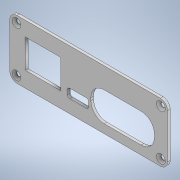
# Autodesk Inventor part: cover-slave
Saved by Autodesk Inventor 2021 (Build 250183000, 183)
## iProperties
Created: 2025-06-25
Part Number: cover-slave
Material: Generic
Document SubType Name: Modeling
Designer: Toby
Density: 1 g/cm^3
Appearance: Default
Author: Toby
Autodesk Inventor part; units mm, degrees
ref_plane "YZ Plane" through (0, 0, 0) normal (1, 0, 0) x (0, 1, 0)
ref_plane "XZ Plane" through (0, 0, 0) normal (0, 1, 0) x (-1, 0, 0)
ref_plane "XY Plane" through (0, 0, 0) normal (0, 0, 1) x (1, 0, 0)
sketch "Sketch1" plane through (0, 0, 0) normal (0, 0, 1) x (1, 0, 0)
  line L0 (-35.5, 13.25) -> (35.5, 13.25)
  line L1 (35.5, 13.25) -> (35.5, -13.25)
  line L2 (35.5, -13.25) -> (-35.5, -13.25)
  line L3 (-35.5, -13.25) -> (-35.5, 13.25)
  point P0 (0, 0)
  dimension "d0" = 26.5
  dimension "d1" = 71
  dimension "d2" = 35.5
  dimension "d3" = 13.25
  constraints: 8 end point, 2 parallel, 1 horizontal, 1 perpendicular
  measures "d0" distance of L2.end L0.start
  measures "d1" distance of L0.start L0.end
  measures "d2" distance from line of point (0, 0) L3
  measures "d3" distance from line of point (0, 0) L0
extrude "Extrusion1" add sketch "Sketch1" along normal blind 1.2
fillet "Fillet1" radius 3.25 4 edges at (-35.5, 13.25, 0.6) (-35.5, -13.25, 0.6) (35.5, -13.25, 0.6) (35.5, 13.25, 0.6)
sketch "Sketch2" plane through (0, 0, 1.2) normal (0, 0, 1) x (1, 0, 0)
  line L0 (32.25, 13.25) -> (-32.25, 13.25) projected
  line L1 (-35.5, 10) -> (-35.5, -10) projected
  line L2 (-32.25, -13.25) -> (32.25, -13.25) projected
  line L3 (35.5, -10) -> (35.5, 10) projected
  point P0 (0, 0)
  point P1 (-32.5, 10.25)
  point P2 (32.5, 10.25)
  point P3 (32.5, -10.25)
  point P4 (-32.5, -10.25)
  dimension "d7" = 3
  dimension "d8" = 3
  dimension "d9" = 3
  dimension "d10" = 3
  dimension "d11" = 3
  dimension "d12" = 3
  dimension "d13" = 3
  dimension "d14" = 3
  measures "d7" distance from line of L0 point (-32.5, 10.25)
  measures "d8" distance from line of L1 point (-32.5, 10.25)
  measures "d9" distance from line of L1 point (-32.5, -10.25)
  measures "d10" distance from line of L2 point (-32.5, -10.25)
  measures "d11" distance from line of L3 point (32.5, -10.25)
  measures "d12" distance from line of L2 point (32.5, -10.25)
  measures "d13" distance from line of L0 point (32.5, 10.25)
  measures "d14" distance from line of L3 point (32.5, 10.25)
hole "Hole1" at (-32.5, 10.25, 1.2) at (32.5, 10.25, 1.2) at (32.5, -10.25, 1.2) at (-32.5, -10.25, 1.2) direction (0, 0, -1) diameter 2 depth 4 tip angle 118 countersink diameter 4 countersink angle 90
sketch "Sketch3" plane through (0, 0, 1.2) normal (0, 0, 1) x (1, 0, 0)
  line L0 (-28.5, 6.75) -> (-12.5, 6.75)
  line L1 (-12.5, 6.75) -> (-12.5, -6.25)
  line L2 (-12.5, -6.25) -> (-28.5, -6.25)
  line L3 (-28.5, -6.25) -> (-28.5, 6.75)
  line L4 (-35.5, 10) -> (-35.5, -10) projected
  line L5 (-32.25, -13.25) -> (32.25, -13.25) projected
  point P0 (0, 0)
  dimension "d22" = 7
  dimension "d23" = 23
  dimension "d24" = 7
  dimension "d25" = 20
  constraints: 8 end point, 2 parallel, 1 horizontal, 1 perpendicular
  measures "d22" distance between parallel lines of L4 L3
  measures "d23" distance between parallel lines of L4 L1
  measures "d24" distance between parallel lines of L5 L2
  measures "d25" distance between parallel lines of L5 L0
extrude "Extrusion2" cut sketch "Sketch3" against normal blind 2
sketch "Sketch4" plane through (0, 0, 1.2) normal (0, 0, 1) x (1, 0, 0)
  line L0 (-9.5, -3.25) -> (0, -3.25)
  line L1 (0, -3.25) -> (0, -7.25)
  line L2 (0, -7.25) -> (-9.5, -7.25)
  line L3 (-9.5, -7.25) -> (-9.5, -3.25)
  line L4 (-35.5, 10) -> (-35.5, -10) projected
  line L5 (-32.25, -13.25) -> (32.25, -13.25) projected
  point P0 (0, 0)
  dimension "d28" = 26
  dimension "d29" = 35.5
  dimension "d30" = 6
  dimension "d31" = 10
  constraints: 8 end point, 2 parallel, 1 horizontal, 1 perpendicular
  measures "d28" distance between parallel lines of L4 L3
  measures "d29" distance between parallel lines of L4 L1
  measures "d30" distance between parallel lines of L5 L2
  measures "d31" distance between parallel lines of L5 L0
extrude "Extrusion3" cut sketch "Sketch4" against normal blind 2
sketch "Sketch5" plane through (0, 0, 1.2) normal (0, 0, 1) x (1, 0, 0)
  line L0 (6.5, 1.75) -> (24.5, 1.75)
  line L1 (24.5, 1.75) -> (24.5, -5.25)
  line L2 (24.5, -5.25) -> (6.5, -5.25)
  line L3 (6.5, -5.25) -> (6.5, 1.75)
  line L4 (35.5, -10) -> (35.5, 10) projected
  line L5 (-32.25, -13.25) -> (32.25, -13.25) projected
  point P0 (0, 0)
  dimension "d34" = 11
  dimension "d35" = 29
  dimension "d36" = 15
  dimension "d37" = 8
  constraints: 8 end point, 2 parallel, 1 horizontal, 1 perpendicular
  measures "d34" distance between parallel lines of L4 L1
  measures "d35" distance between parallel lines of L4 L3
  measures "d36" distance between parallel lines of L5 L0
  measures "d37" distance between parallel lines of L5 L2
extrude "Extrusion4" cut sketch "Sketch5" against normal blind 2
chamfer "Chamfer1" distance 2 angle 45 2 edges at (6.5, -5.25, 0.6) (24.5, -5.25, 0.6)
fillet "Fillet2" radius 1 4 edges at (-9.5, -3.25, 0.6) (-9.5, -7.25, 0.6) (0, -7.25, 0.6) (0, -3.25, 0.6)
sketch "Sketch7" plane through (0, 0, 1.2) normal (0, 0, 1) x (1, 0, 0)
  line L0 (1, 3.85) -> (29.6, 3.85)
  line L1 (29.6, 3.85) -> (29.6, -9.35)
  line L2 (29.6, -9.35) -> (1, -9.35)
  line L3 (1, -9.35) -> (1, 3.85)
  line L4 (-32.25, -13.25) -> (32.25, -13.25) projected
  line L5 (35.5, -10) -> (35.5, 10) projected
  point P0 (0, 0)
  dimension "d56" = 3.9
  dimension "d57" = 5.9
  dimension "d58" = 17.1
  dimension "d59" = 34.5
  constraints: 8 end point, 2 parallel, 1 horizontal, 1 perpendicular
  measures "d56" distance between parallel lines of L4 L2
  measures "d57" distance between parallel lines of L5 L1
  measures "d58" distance between parallel lines of L4 L0
  measures "d59" distance between parallel lines of L5 L3
extrude "Extrusion6" cut sketch "Sketch7" against normal blind 2
fillet "Fillet3" radius 6 4 edges at (1, 3.85, 0.6) (1, -9.35, 0.6) (29.6, 3.85, 0.6) (29.6, -9.35, 0.6)
body "Solid1"
